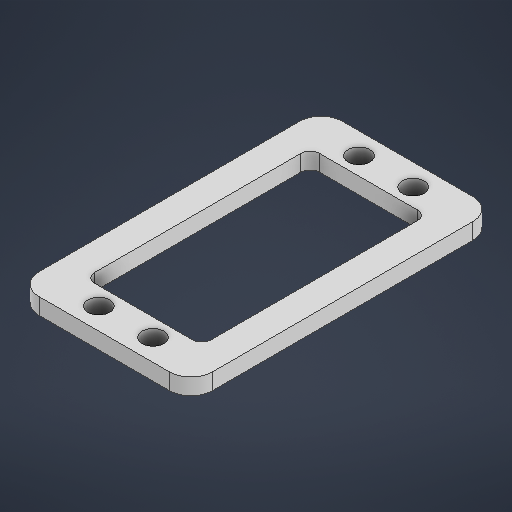
# Autodesk Inventor part: ClawServoPlate
Saved by Autodesk Inventor 2025 (Build 290162000, 162)
## iProperties
Created: 2024-05-20
Part Number: ClawServoPlate
Material: Generic
Document SubType Name: Modeling
Designer: avsar
Density: 1 g/cm^3
Appearance: Default
Author: avsar
Autodesk Inventor part; units mm, degrees
ref_plane "YZ Plane" through (0, 0, 0) normal (1, 0, 0) x (0, 1, 0)
ref_plane "XZ Plane" through (0, 0, 0) normal (0, 1, 0) x (-1, 0, 0)
ref_plane "XY Plane" through (0, 0, 0) normal (0, 0, 1) x (1, 0, 0)
sketch "Sketch1" plane through (0, 0, 0) normal (0, 1, 0) x (-1, 0, 0)
  line L0 (9, 20.5) -> (-9, 20.5) construction
  line L1 (-10.5, 19) -> (-10.5, -19) construction
  line L2 (-9, -20.5) -> (9, -20.5) construction
  line L3 (10.5, -19) -> (10.5, 19) construction
  line L4 (10.5, 20.5) -> (-10.5, -20.5) construction
  line L5 (-10.5, 20.5) -> (10.5, -20.5) construction
  circle A0 centre (-5, 24) radius 2
  line L6 (0, 0) -> (10.5, 0) construction
  line L7 (0, 0) -> (0, -20.5) construction
  circle A1 centre (5, 24) radius 2
  circle A2 centre (-5, -24) radius 2
  circle A3 centre (5, -24) radius 2
  arc A4 (9, -20.5) -> (10.5, -19) centre (9, -19) ccw
  arc A5 (-10.5, -19) -> (-9, -20.5) centre (-9, -19) ccw construction
  arc A6 (10.5, 19) -> (9, 20.5) centre (9, 19) ccw
  arc A7 (-9, 20.5) -> (-10.5, 19) centre (-9, 19) ccw construction
  line L8 (9, -20.75) -> (-9, -20.75)
  arc A8 (-10.75, -19) -> (-9, -20.75) centre (-9, -19) ccw
  line L9 (-10.75, -19) -> (-10.75, 19)
  arc A9 (-9, 20.75) -> (-10.75, 19) centre (-9, 19) ccw
  line L10 (-9, 20.75) -> (9, 20.75)
  arc A10 (10.75, 19) -> (9, 20.75) centre (9, 19) ccw
  line L11 (10.75, 19) -> (10.75, -19)
  arc A11 (9, -20.75) -> (10.75, -19) centre (9, -19) ccw
  line L12 (16, -28) -> (-16, -28)
  line L13 (-16, -28) -> (-16, 28)
  line L14 (-16, 28) -> (16, 28)
  line L15 (16, 28) -> (16, -28)
  line L16 (16, -28) -> (-16, 28) construction
  line L17 (-16, -28) -> (16, 28) construction
  line L18 (-12.5, -12) -> (-12.5, 12) construction
  point P0 (-12.5, 0)
  dimension "d0" = 21
  dimension "d1" = 41
  dimension "d2" = 4
  dimension "d3" = 5
  dimension "d4" = 24
  dimension "d5" = 1.5
  dimension "d6" = 0.25
  dimension "d7" = 32
  dimension "d8" = 56
  dimension "d12" = 24
  dimension "d13" = 3.5
  dimension "d16" = 0
  constraints: 38 end point, 16 point on circle, 12 centre point, 8 point on line, 8 tangent, 7 midpoint, 6 parallel, 3 equal radius, 3 perpendicular, 3 symmetric about line, 2 horizontal, 1 coincident, 1 horizontal alignment, 1 vertical, 1 vertical alignment, 10 other
  measures "d0" distance of L5.end L4.end
  measures "d1" distance of L4.end L5.start
  measures "d2" diameter of A0
  measures "d3" horizontal distance of L6.start A0.centre
  measures "d4" vertical distance of L6.start A0.centre
  measures "d5" radius of A4
  measures "d6" distance between parallel lines of L2 L8
  measures "d7" distance of L13.end L14.end
  measures "d8" distance of L12.end L13.end
  measures "d12" distance of L18.start L18.end
  measures "d13" distance from line of L13 L18.start
  measures "d16" distance of L6.start point (0, 0)
extrude "Extrusion1" add sketch "Sketch1" along normal blind 3
fillet "Fillet1" radius 4 4 edges at (16, 1.5, 28) (-16, 1.5, 28) (16, 1.5, -28) (-16, 1.5, -28)
body "Solid1"
